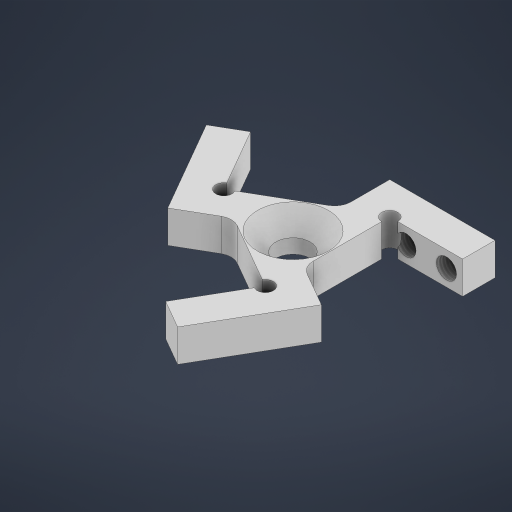
# Autodesk Inventor part: ServoCap
Saved by Autodesk Inventor 2023 (Build 270158000, 158)
## iProperties
Created: 2023-02-25
Part Number: ServoCap
Material: Generic
Document SubType Name: Modeling
Designer: roota
Density: 1 g/cm^3
Appearance: Default
Author: roota
Autodesk Inventor part; units mm, degrees
ref_plane "YZ Plane" through (0, 0, 0) normal (1, 0, 0) x (0, 1, 0)
ref_plane "XZ Plane" through (0, 0, 0) normal (0, 1, 0) x (-1, 0, 0)
ref_plane "XY Plane" through (0, 0, 0) normal (0, 0, 1) x (1, 0, 0)
sketch "Sketch1" plane through (0, 0, 0) normal (0, 1, 0) x (-1, 0, 0)
  line L0 (-0.9998, -14.9003) -> (-26.9998, -14.9003)
  line L1 (-26.9998, -14.9003) -> (-26.9998, -22.9003)
  line L2 (-26.9998, -22.9003) -> (-0.9998, -22.9003)
  line L3 (-0.9998, -22.9003) -> (-0.9998, -14.9003)
  line L4 (-0.9998, -14.9003) -> (-8.9998, -14.9003)
  line L5 (-8.9998, -14.9003) -> (-8.9998, -10.9694)
  line L6 (-8.9998, -10.9694) -> (-0.9998, -10.9694) construction
  line L7 (-0.9998, -10.9694) -> (-0.9998, -14.9003)
  line L8 (13.404, 6.5843) -> (26.404, -15.9324)
  line L9 (26.404, -15.9324) -> (33.3322, -11.9324)
  line L10 (33.3322, -11.9324) -> (20.3322, 10.5843)
  line L11 (20.3322, 10.5843) -> (13.404, 6.5843)
  line L12 (13.404, 6.5843) -> (17.404, -0.3439)
  line L13 (17.404, -0.3439) -> (13.9997, -2.3094)
  line L14 (13.9997, -2.3094) -> (9.9997, 4.6188) construction
  line L15 (9.9997, 4.6188) -> (13.404, 6.5843)
  line L16 (-12.4041, 8.316) -> (0.5959, 30.8327)
  line L17 (0.5959, 30.8327) -> (-6.3323, 34.8327)
  line L18 (-6.3323, 34.8327) -> (-19.3323, 12.316)
  line L19 (-19.3323, 12.316) -> (-12.4041, 8.316)
  line L20 (-12.4041, 8.316) -> (-8.4041, 15.2442)
  line L21 (-8.4041, 15.2442) -> (-4.9998, 13.2788)
  line L22 (-4.9998, 13.2788) -> (-8.9998, 6.3506) construction
  line L23 (-8.9998, 6.3506) -> (-12.4041, 8.316)
  line L24 (17.9997, 0) -> (-8.9998, -15.5882)
  line L25 (-8.9998, -15.5882) -> (-8.9998, 15.5882)
  line L26 (-8.9998, 15.5882) -> (17.9997, 0)
  point P0 (0, 0)
  point P1 (0, 0)
  point P2 (17.404, -0.3439)
  dimension "d0" = 8
  dimension "d3" = 360
  dimension "d5" = 60.332
  dimension "d6" = 57.733
  dimension "d7" = 26
  constraints: 54 end point, 4 parallel, 3 perpendicular, 2 horizontal, 2 point on line, 1 coincident, 1 vertical, 53 other
  measures "d0" distance of L1.end L0.end
  measures "d5" distance from line of L1 L9.end
  measures "d6" distance from line of L17.end L2
  measures "d7" distance of L1.end L2.end
extrude "Extrusion1" add sketch "Sketch1" along normal blind 8
fillet "Fillet1" radius 4 3 edges at (8.9998, 4, 6.3506) (-9.9997, 4, 4.6188) (0.9998, 4, -10.9694)
sketch "Sketch2" plane through (0, 8, 0) normal (0, 1, 0) x (1, 0, 0)
  line L0 (8.9998, -4.0412) -> (8.9998, 14.9003) projected
  circle A0 centre (8.9998, 14.9003) radius 2
  line L1 (8.4041, -15.2442) -> (-0.5959, -30.8327) projected
  circle A1 centre (8.4041, -15.2442) radius 2
  line L2 (-1.0002, 9.8147) -> (-17.404, 0.3439) projected
  circle A2 centre (-17.404, 0.3439) radius 2
  circle A3 centre (0, 0) radius 4.25
  dimension "d11" = 4
  dimension "d14" = 8.5
  constraints: 4 centre point, 2 equal radius, 1 coincident
  measures "d11" diameter of A0
  measures "d14" diameter of A3
extrude "Extrusion2" cut sketch "Sketch2" against normal blind 18.75
chamfer "Chamfer1" distance 4.5 angle 45 1 edges at (-4.25, 8, 0)
sketch "Sketch3" plane through (26.9998, 0, -22.9003) normal (0, 0, -1) x (-1, 0, 0)
  circle A0 centre (4, 4) radius 2.5
  circle A1 centre (14, 4) radius 2.5
  line L0 (0, 0) -> (26, 0) projected
  line L1 (0, 0) -> (0, 8) projected
  point P0 (26.9998, 0)
  dimension "d18" = 10
  dimension "d19" = 5
  dimension "d20" = 4
  dimension "d21" = 4
  constraints: 2 centre point, 1 equal radius, 1 horizontal alignment
  measures "d18" distance of A0.centre A1.centre
  measures "d19" diameter of A0
  measures "d20" distance from line of L0 A0.centre
  measures "d21" distance from line of A0.centre L1
extrude "Extrusion3" cut sketch "Sketch3" against normal blind 18.75
thread "Thread1" size "M5x0.8" class "6H" standard "ISO Metric profile" length 15
thread "Thread2" size "M5x0.8" class "6H" standard "ISO Metric profile" length 15
body "Solid1"
